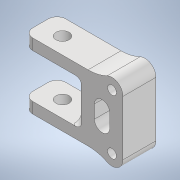
# Autodesk Inventor part: 2020_fixer_1
Saved by Autodesk Inventor 2020 (Build 240168000, 168)
## iProperties
Created: 2019-10-23
Part Number: 2020_fixer_1
Material: Generic
Document SubType Name: Modeling
Designer: psrob
Density: 1 g/cm^3
Appearance: Default
Author: psrob
Autodesk Inventor part; units mm, degrees
ref_plane "YZ Plane" through (0, 0, 0) normal (1, 0, 0) x (0, 1, 0)
ref_plane "XZ Plane" through (0, 0, 0) normal (0, 1, 0) x (-1, 0, 0)
ref_plane "XY Plane" through (0, 0, 0) normal (0, 0, 1) x (1, 0, 0)
sketch "Sketch1" plane through (0, 0, 0) normal (0, 0, 1) x (1, 0, 0)
  circle A0 centre (19.8085, -5.5) radius 1 projected
  circle A1 centre (30.8085, -5.5) radius 1 projected
  circle A2 centre (19.8085, 5.5) radius 1 projected
  circle A3 centre (30.8085, 5.5) radius 1 projected
  circle A4 centre (25.3085, 0) radius 6.65 projected
  line L0 (41.3085, 2) -> (41.3085, -2) projected
  line L1 (35.1065, 2) -> (41.3085, 2) projected
  arc A5 (35.1065, 2) -> (26.5426, 9.9236) centre (25.3085, 0) ccw projected
  line L2 (26.5426, 9.9236) -> (-34.0744, 17.4618) projected
  arc A6 (-34.0744, 17.4618) -> (-39.6915, 12.5) centre (-34.6915, 12.5) ccw projected
  line L3 (-39.6915, 12.5) -> (-39.6915, -12.5) projected
  arc A7 (-39.6915, -12.5) -> (-34.0744, -17.4618) centre (-34.6915, -12.5) ccw projected
  line L4 (-34.0744, -17.4618) -> (26.5426, -9.9236) projected
  arc A8 (26.5426, -9.9236) -> (35.1065, -2) centre (25.3085, 0) ccw projected
  line L5 (41.3085, -2) -> (35.1065, -2) projected
  circle A9 centre (-34.6915, 12.5) radius 2 projected
  circle A10 centre (-34.6915, -12.5) radius 2 projected
  line L6 (-25.1979, 6.2809) -> (9.3489, 1.9847) projected
  arc A11 (9.3489, -1.9847) -> (9.3489, 1.9847) centre (9.1021, 0) ccw projected
  line L7 (9.3489, -1.9847) -> (-25.1979, -6.2809) projected
  arc A12 (-29.6915, -2.3115) -> (-25.1979, -6.2809) centre (-25.6915, -2.3115) ccw projected
  line L8 (-29.6915, -2.3115) -> (-29.6915, 2.3115) projected
  arc A13 (-25.1979, 6.2809) -> (-29.6915, 2.3115) centre (-25.6915, 2.3115) ccw projected
  circle A14 centre (-34.6915, -12.5) radius 5
  circle A15 centre (-34.6915, 12.5) radius 5
  line L9 (-34.6915, -12.5) -> (-34.6915, 12.5)
  line L10 (-34.6915, -12.5) -> (-29.6915, -12.5)
  line L11 (-34.6915, 12.5) -> (-29.6915, 12.5)
  line L12 (-29.6915, 12.5) -> (-29.6915, -12.5)
  line L13 (-34.6915, 0) -> (-64.6915, 0)
  line L14 (-64.6915, -10) -> (-64.6915, 10)
  line L15 (-64.6915, 10) -> (-34.6915, 10)
  line L16 (-34.6915, 10) -> (-34.6915, -10)
  line L17 (-34.6915, -10) -> (-64.6915, -10)
  line L18 (-64.6915, -10) -> (-34.6915, 10) construction
  line L19 (-64.6915, 10) -> (-34.6915, -10) construction
  line L20 (-64.6915, -10) -> (-34.6915, -10)
  line L21 (-34.6915, -10) -> (-34.6915, -15)
  line L22 (-34.6915, -15) -> (-64.6915, -15)
  line L23 (-64.6915, -15) -> (-64.6915, -10)
  line L24 (-64.6915, 10) -> (-34.6915, 10)
  line L25 (-34.6915, 10) -> (-34.6915, 15)
  line L26 (-34.6915, 15) -> (-64.6915, 15)
  line L27 (-64.6915, 15) -> (-64.6915, 10)
  point P0 (0, 0)
  point P1 (-49.6915, 0)
  point P2 (-39.0216, 15)
  point P3 (-39.6915, 10)
  point P4 (-39.6915, -10)
  point P5 (-39.0216, -15)
  dimension "d0" = 10
  dimension "d1" = 10
  dimension "d2" = 30
  dimension "d3" = 20
  dimension "d4" = 30
  dimension "d5" = 30
  dimension "d6" = 5
  dimension "d7" = 30
  dimension "d8" = 5
  constraints: 38 end point, 7 parallel, 4 horizontal, 4 midpoint, 4 perpendicular, 2 coincident, 1 vertical, 6 other
  measures "d2" distance of L13.start L13.end
  measures "d3" distance of L14.start L14.end
  measures "d4" distance of L14.end L15.end
  measures "d5" distance of L21.end L22.end
  measures "d6" distance of L20.end L21.end
  measures "d7" distance of L26.end L25.end
  measures "d8" distance of L25.end L24.end
extrude "Extrusion1" add sketch "Sketch1" along normal blind 10 contours A15 L11 A9 L25 L26 A6 | A7 L22 L21 A10 L10 A14 | L26 L25 A9 L9 L15 A15 A6 | A6 L3 L15 L27 L26 | L12 L8 A14 L9 A15 | A15 L9 A9 L11 | L22 L23 L17 L3 A7 | A7 A14 L17 L9 A10 L21 L22 | L10 A10 L9 A14 | A15 L15 L3 | L9 L13 L3 L15 A15 | A15 L15 L9 | L3 L17 A14 | L9 L17 A14 | A14 L17 L3 L13 L9
thicken "Thicken1" operation add thickness 10 both sides no extend neighbours yes toward (-1, 0, 0) faces at (-64.6915, -11.6667, 3.3333)
thicken "Thicken2" operation add thickness 10 both sides no extend neighbours yes toward (-1, 0, 0) faces at (-64.6915, 13.3333, 3.3333)
sketch "Sketch2" plane through (0, 0, 10) normal (0, 0, 1) x (1, 0, 0)
  line L0 (-39.6915, 10) -> (-39.6915, -10) projected
  line L1 (-39.6915, -10) -> (-74.6915, -10) projected
  line L2 (-74.6915, -10) -> (-74.6915, -15) projected
  line L3 (-74.6915, -15) -> (-39.0216, -15) projected
  arc A0 (-39.0216, -15) -> (-29.6915, -12.5) centre (-34.6915, -12.5) ccw projected
  line L4 (-29.6915, -12.5) -> (-29.6915, 12.5) projected
  arc A1 (-29.6915, 12.5) -> (-39.0216, 15) centre (-34.6915, 12.5) ccw projected
  line L5 (-39.0216, 15) -> (-74.6915, 15) projected
  line L6 (-74.6915, 15) -> (-74.6915, 10) projected
  line L7 (-74.6915, 10) -> (-39.6915, 10) projected
  circle A2 centre (-34.6915, -12.5) radius 2 projected
  circle A3 centre (-34.6915, 12.5) radius 2 projected
  point P0 (0, 0)
extrude "Extrusion2" add sketch "Sketch2" along normal blind 5
sketch "Sketch3" plane through (0, 0, 15) normal (0, 0, 1) x (1, 0, 0)
  line L0 (-39.6915, 10) -> (-39.6915, -10) projected
  line L1 (-39.6915, -10) -> (-74.6915, -10) projected
  line L2 (-74.6915, -10) -> (-74.6915, -15) projected
  line L3 (-74.6915, -15) -> (-39.0216, -15) projected
  arc A0 (-39.0216, -15) -> (-29.6915, -12.5) centre (-34.6915, -12.5) ccw projected
  line L4 (-29.6915, -12.5) -> (-29.6915, 12.5) projected
  arc A1 (-29.6915, 12.5) -> (-39.0216, 15) centre (-34.6915, 12.5) ccw projected
  line L5 (-39.0216, 15) -> (-74.6915, 15) projected
  line L6 (-74.6915, 15) -> (-74.6915, 10) projected
  line L7 (-74.6915, 10) -> (-39.6915, 10) projected
  circle A2 centre (-34.6915, -12.5) radius 2 projected
  circle A3 centre (-34.6915, 12.5) radius 2 projected
  line L8 (-39.6915, 10) -> (-39.6915, -10) projected
  line L9 (-39.6915, 10) -> (-52.6915, 10)
  line L10 (-52.6915, 10) -> (-52.6915, -10)
  line L11 (-52.6915, -10) -> (-39.6915, -10)
  line L12 (-39.6915, -10) -> (-39.6915, 10)
  point P0 (0, 0)
  dimension "d17" = 13
  dimension "d18" = 20
  constraints: 8 end point, 2 parallel, 1 horizontal, 1 perpendicular
  measures "d17" distance of L11.end L10.end
  measures "d18" distance of L10.end L9.end
extrude "Extrusion3" add sketch "Sketch3" against normal up to surface (15 mm away) contours L0 L1 L10 L7
chamfer "Chamfer1" distance 4 angle 45 2 edges at (-52.6915, 0, 0) (-52.6915, 0, 15)
fillet "Fillet1" radius 20 2 edges at (-39.0216, -15, 7.5) (-39.0216, 15, 7.5)
sketch "Sketch4" plane through (0, 0, 15) normal (0, 0, 1) x (1, 0, 0)
  line L0 (-48.6915, -10) -> (-74.6915, -10) projected
  line L1 (-74.6915, -10) -> (-74.6915, -15) projected
  line L2 (-74.6915, -15) -> (-45.5887, -15) projected
  arc A0 (-36.8709, -17) -> (-45.5887, -15) centre (-45.5887, -35) ccw projected
  arc A1 (-36.8709, -17) -> (-29.6915, -12.5) centre (-34.6915, -12.5) ccw projected
  line L3 (-29.6915, -12.5) -> (-29.6915, 12.5) projected
  arc A2 (-29.6915, 12.5) -> (-36.8709, 17) centre (-34.6915, 12.5) ccw projected
  arc A3 (-45.5887, 15) -> (-36.8709, 17) centre (-45.5887, 35) ccw projected
  line L4 (-45.5887, 15) -> (-74.6915, 15) projected
  line L5 (-74.6915, 15) -> (-74.6915, 10) projected
  line L6 (-74.6915, 10) -> (-48.6915, 10) projected
  line L7 (-48.6915, -10) -> (-48.6915, 10) projected
  circle A4 centre (-34.6915, -12.5) radius 2 projected
  circle A5 centre (-34.6915, 12.5) radius 2 projected
  circle A6 centre (-34.6915, -12.5) radius 2 projected
  line L8 (-34.6915, 12.5) -> (-34.6915, -12.5)
  line L9 (-34.6915, 0) -> (-39.1915, 0)
  line L10 (-39.1915, 3) -> (-39.1915, -3) construction
  line L11 (-42.6915, 3) -> (-42.6915, -3)
  line L12 (-35.6915, -3) -> (-35.6915, 3)
  arc A7 (-35.6915, 3) -> (-42.6915, 3) centre (-39.1915, 3) ccw
  arc A8 (-42.6915, -3) -> (-35.6915, -3) centre (-39.1915, -3) ccw
  point P0 (0, 0)
  dimension "d25" = 4.5
  dimension "d26" = 3
  dimension "d27" = 7
  constraints: 12 end point, 4 point on circle, 4 tangent, 2 centre point, 2 midpoint, 1 horizontal, 1 parallel, 1 perpendicular, 1 vertical
  measures "d25" distance of L9.start L9.end
  measures "d26" distance of L9.end L10.end
  measures "d27" diameter of A8
extrude "Extrusion4" cut sketch "Sketch4" against normal blind 20 contours A7 L12 A8 L11
sketch "Sketch5" plane through (-74.6915, -15, 0) normal (0, -1, 0) x (1, 0, 0)
  line L0 (29.1028, 15) -> (29.1028, 0) projected
  line L1 (0, 15) -> (29.1028, 15) projected
  line L2 (0, 0) -> (0, 15) projected
  line L3 (0, 0) -> (29.1028, 0) projected
  line L4 (0, 0) -> (0, 15) projected
  line L5 (0, 7.5) -> (10, 7.5)
  circle A0 centre (10, 7.5) radius 3
  point P0 (74.6915, 0)
  dimension "d30" = 10
  dimension "d31" = 6
  constraints: 2 end point, 1 centre point, 1 coincident, 1 horizontal, 1 midpoint
  measures "d30" distance of L5.start L5.end
  measures "d31" diameter of A0
extrude "Extrusion5" cut sketch "Sketch5" against normal blind 30 contours A0
fillet "Fillet2" radius 2 4 edges at (-50.6915, 10, 13) (-50.6915, -10, 13) (-50.6915, -10, 2) (-50.6915, 10, 2)
fillet "Fillet3" radius 4 4 edges at (-74.6915, -12.5, 0) (-74.6915, -12.5, 15) (-74.6915, 12.5, 0) (-74.6915, 12.5, 15)
body "Solid1"
